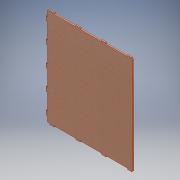
# Autodesk Inventor part: Base
Saved by Autodesk Inventor 2017 (Build 210142000, 142)
## iProperties
Created: 2017-10-03
Part Number: Base
Material: Wood (Oak)
Document SubType Name: Modeling
Designer: Felipe
Density: 0.76 g/cm^3
Appearance: White Oak - Natural Medium Gloss
Author: Felipe
Autodesk Inventor part; units mm, degrees
ref_plane "YZ Plane" through (0, 0, 0) normal (1, 0, 0) x (0, 1, 0)
ref_plane "XZ Plane" through (0, 0, 0) normal (0, 1, 0) x (-1, 0, 0)
ref_plane "XY Plane" through (0, 0, 0) normal (0, 0, 1) x (1, 0, 0)
sketch "Sketch1" plane through (0, 0, 0) normal (0, 1, 0) x (-1, 0, 0)
  line L0 (0, 0) -> (792, 0) construction
  line L1 (792, 0) -> (792, -900) construction
  line L2 (792, -900) -> (0, -900) construction
  line L3 (0, -900) -> (0, 0)
  line L4 (770, 0) -> (730, 0) construction
  line L5 (730, 0) -> (730, 10)
  line L6 (730, 10) -> (770, 10)
  line L7 (770, 10) -> (770, 0)
  line L8 (530, 0) -> (490, 0) construction
  line L9 (490, 0) -> (490, 10)
  line L10 (490, 10) -> (530, 10)
  line L11 (530, 10) -> (530, 0)
  line L12 (290, 0) -> (250, 0) construction
  line L13 (250, 0) -> (250, 10)
  line L14 (250, 10) -> (290, 10)
  line L15 (290, 10) -> (290, 0)
  line L16 (50, 0) -> (10, 0) construction
  line L17 (10, 0) -> (10, 10)
  line L18 (10, 10) -> (50, 10)
  line L19 (50, 10) -> (50, 0)
  line L20 (0, 0) -> (10, 0)
  line L21 (250, 0) -> (50, 0)
  line L22 (490, 0) -> (290, 0)
  line L23 (730, 0) -> (530, 0)
  line L24 (792, 0) -> (770, 0)
  line L25 (792, -450) -> (0, -450) construction
  line L26 (0, -900) -> (792, -900) construction
  line L27 (770, -900) -> (730, -900) construction
  line L28 (730, -900) -> (730, -910)
  line L29 (730, -910) -> (770, -910)
  line L30 (770, -910) -> (770, -900)
  line L31 (530, -900) -> (490, -900) construction
  line L32 (490, -900) -> (490, -910)
  line L33 (490, -910) -> (530, -910)
  line L34 (530, -910) -> (530, -900)
  line L35 (290, -900) -> (250, -900) construction
  line L36 (250, -900) -> (250, -910)
  line L37 (250, -910) -> (290, -910)
  line L38 (290, -910) -> (290, -900)
  line L39 (50, -900) -> (10, -900) construction
  line L40 (10, -900) -> (10, -910)
  line L41 (10, -910) -> (50, -910)
  line L42 (50, -910) -> (50, -900)
  line L43 (0, -900) -> (10, -900)
  line L44 (250, -900) -> (50, -900)
  line L45 (490, -900) -> (290, -900)
  line L46 (730, -900) -> (530, -900)
  line L47 (792, -900) -> (770, -900)
  line L48 (792, -50) -> (805.7739, -50)
  line L49 (805.7739, -50) -> (805.7739, -90)
  line L50 (805.7739, -90) -> (792, -90)
  line L51 (792, -90) -> (792, -50) construction
  line L52 (805.7739, -240) -> (792, -240)
  line L53 (792, -240) -> (792, -280) construction
  line L54 (792, -280) -> (805.7739, -280)
  line L55 (805.7739, -280) -> (805.7739, -240)
  line L56 (805.7739, -430) -> (792, -430)
  line L57 (792, -430) -> (792, -470) construction
  line L58 (792, -470) -> (805.7739, -470)
  line L59 (805.7739, -470) -> (805.7739, -430)
  line L60 (805.7739, -620) -> (792, -620)
  line L61 (792, -620) -> (792, -660) construction
  line L62 (792, -660) -> (805.7739, -660)
  line L63 (805.7739, -660) -> (805.7739, -620)
  line L64 (805.7739, -810) -> (792, -810)
  line L65 (792, -810) -> (792, -850) construction
  line L66 (792, -850) -> (805.7739, -850)
  line L67 (805.7739, -850) -> (805.7739, -810)
  line L68 (792, -850) -> (792, -900)
  line L69 (792, -810) -> (792, -660)
  line L70 (792, -620) -> (792, -470)
  line L71 (792, -430) -> (792, -280)
  line L72 (792, -240) -> (792, -90)
  line L73 (792, -50) -> (792, 0)
  dimension "d0" = 900
  dimension "d1" = 792
  dimension "d2" = 40
  dimension "d3" = 22
  dimension "d4" = 10
  dimension "d5" = 200
  dimension "d6" = 200
  dimension "d9" = 200
  dimension "d12" = 50
  dimension "d13" = 40
  dimension "d14" = 150
  dimension "d15" = 150
  dimension "d16" = 150
  dimension "d17" = 150
  dimension "d18" = 50
  constraints: 148 end point, 23 point on line, 20 parallel, 16 symmetric about line, 14 collinear, 13 horizontal, 11 perpendicular, 2 midpoint
  measures "d0" distance of L0.end L1.end
  measures "d1" distance of L0.start L0.end
  measures "d2" distance of L5.end L6.end
  measures "d3" distance between parallel lines of L1 L7
  measures "d4" distance of L6.end L4.start
  measures "d5" distance between parallel lines of L11 L5
  measures "d6" distance from line of L19 L12.end
  measures "d9" distance between parallel lines of L15 L9
  measures "d12" distance between parallel lines of L48 L0
  measures "d13" distance of L48.end L49.end
  measures "d14" distance between parallel lines of L52 L50
  measures "d15" distance between parallel lines of L56 L54
  measures "d16" distance between parallel lines of L60 L58
  measures "d17" distance between parallel lines of L64 L62
  measures "d18" distance between parallel lines of L2 L66
extrude "Extrusion1" add sketch "Sketch1" along normal blind 10
body "Solid1"
